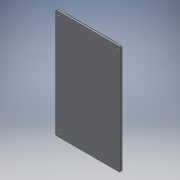
# Autodesk Inventor part: Tampa caixa principal
Saved by Autodesk Inventor 2019 (Build 230136000, 136)
## iProperties
Created: 2020-06-01
Part Number: Tampa caixa principal
Material: Generic
Document SubType Name: Modeling
Designer: luiza
Density: 1 g/cm^3
Appearance: Default
Author: luiza
Autodesk Inventor part; units mm, degrees
ref_plane "YZ Plane" through (0, 0, 0) normal (1, 0, 0) x (0, 1, 0)
ref_plane "XZ Plane" through (0, 0, 0) normal (0, 1, 0) x (-1, 0, 0)
ref_plane "XY Plane" through (0, 0, 0) normal (0, 0, 1) x (1, 0, 0)
sketch "Sketch1" plane through (0, 0, 0) normal (0, 0, 1) x (1, 0, 0)
  circle A0 centre (50, 87.5) radius 2.01 projected
  circle A1 centre (50, -87.5) radius 2.01 projected
  line L0 (55, -90.5) -> (55, 90.5) projected
  arc A2 (55, 90.5) -> (53, 92.5) centre (53, 90.5) ccw projected
  line L1 (53, 92.5) -> (-53, 92.5) projected
  arc A3 (-53, 92.5) -> (-55, 90.5) centre (-53, 90.5) ccw projected
  line L2 (-55, 90.5) -> (-55, -90.5) projected
  arc A4 (-55, -90.5) -> (-53, -92.5) centre (-53, -90.5) ccw projected
  line L3 (-53, -92.5) -> (53, -92.5) projected
  arc A5 (53, -92.5) -> (55, -90.5) centre (53, -90.5) ccw projected
  circle A6 centre (-50, 87.5) radius 2.01 projected
  circle A7 centre (-50, -87.5) radius 2.01 projected
ref_plane "Work Plane1" through (0, 0, 0) normal (0, 0, -1) x (-1, 0, 0)
sketch "Sketch2" plane through (0, 0, 0) normal (0, 0, -1) x (-1, 0, 0)
  arc A0 (42.8653, 89.5) -> (52, 80.3653) centre (55, 92.5) ccw projected
  line L0 (42.8653, 89.5) -> (-42.8653, 89.5) projected
  arc A1 (-52, 80.3653) -> (-42.8653, 89.5) centre (-55, 92.5) ccw projected
  line L1 (-52, 80.3653) -> (-52, -80.3653) projected
  line L2 (52, -80.3653) -> (52, 80.3653) projected
  arc A2 (52, -80.3653) -> (42.8653, -89.5) centre (55, -92.5) ccw projected
  line L3 (-42.8653, -89.5) -> (42.8653, -89.5) projected
  arc A3 (-42.8653, -89.5) -> (-52, -80.3653) centre (-55, -92.5) ccw projected
  line L4 (-42.4044, 88.9) -> (42.4044, 88.9)
  arc A4 (42.4044, 88.9) -> (51.4, 79.9044) centre (55, 92.5) ccw
  line L5 (51.4, 79.9044) -> (51.4, -79.9044)
  arc A5 (51.4, -79.9044) -> (42.4044, -88.9) centre (55, -92.5) ccw
  line L6 (42.4044, -88.9) -> (-42.4044, -88.9)
  arc A6 (-42.4044, -88.9) -> (-51.4, -79.9044) centre (-55, -92.5) ccw
  line L7 (-51.4, -79.9044) -> (-51.4, 79.9044)
  arc A7 (-51.4, 79.9044) -> (-42.4044, 88.9) centre (-55, 92.5) ccw
  line L8 (39.6817, 84.9) -> (-39.6817, 84.9)
  arc A8 (-47.4, 77.1817) -> (-39.6817, 84.9) centre (-55, 92.5) ccw
  line L9 (-47.4, 77.1817) -> (-47.4, -77.1817)
  arc A9 (-39.6817, -84.9) -> (-47.4, -77.1817) centre (-55, -92.5) ccw
  line L10 (-39.6817, -84.9) -> (39.6817, -84.9)
  arc A10 (47.4, -77.1817) -> (39.6817, -84.9) centre (55, -92.5) ccw
  line L11 (47.4, -77.1817) -> (47.4, 77.1817)
  arc A11 (39.6817, 84.9) -> (47.4, 77.1817) centre (55, 92.5) ccw
  point P0 (-50, -92.5)
  point P1 (50, -92.5)
  point P2 (50, 92.5)
  point P3 (-50, 92.5)
  dimension "d11" = 0.6
  dimension "d12" = 4
  constraints: 16 end point, 16 point on circle, 8 centre point, 14 other
  measures "d11" distance between parallel lines of L0 L4
  measures "d12" distance between parallel lines of L4 L8
extrude "Extrusion2" add sketch "Sketch2" along normal blind 4 contours L4 A4 L5 A5 L6 A6 L7 A7
extrude "Extrusion3" add sketch "Sketch1" along normal blind 3
body "Solid1"
